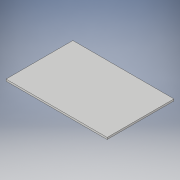
# Autodesk Inventor part: basic side
Saved by Autodesk Inventor 2018 (Build 220112000, 112)
## iProperties
Created: 2018-05-14
Part Number: basic side
Material: Generic
Document SubType Name: Modeling
Designer: Administrator
Density: 1 g/cm^3
Appearance: Default
Author: Administrator
Autodesk Inventor part; units mm, degrees
ref_plane "YZ Plane" through (0, 0, 0) normal (1, 0, 0) x (0, 1, 0)
ref_plane "XZ Plane" through (0, 0, 0) normal (0, 1, 0) x (-1, 0, 0)
ref_plane "XY Plane" through (0, 0, 0) normal (0, 0, 1) x (1, 0, 0)
sketch "Sketch1" plane through (0, 0, 0) normal (0, 0, 1) x (1, 0, 0)
  line L0 (0, 0) -> (355.6, 0)
  line L1 (355.6, 0) -> (355.6, 152.4)
  line L2 (355.6, 152.4) -> (0, 152.4)
  line L3 (0, 152.4) -> (0, 0)
  circle A0 centre (177.8, 76.2) radius 12.7
  circle A1 centre (279.4, 76.2) radius 12.7
  circle A2 centre (76.2, 76.2) radius 12.7
  dimension "d2" = 25.4
  dimension "d3" = 25.4
  dimension "d5" = 25.4
  dimension "d8" = 355.6
  dimension "d9" = 152.4
  dimension "d10" = 101.6
  dimension "d11" = 101.6
  constraints: 8 end point, 3 centre point, 2 parallel, 1 horizontal, 1 perpendicular
  measures "d2" diameter of A0
  measures "d3" diameter of A1
  measures "d5" diameter of A2
  measures "d8" distance of L1.end L2.end
  measures "d9" distance of L0.end L1.end
  measures "d10" distance of A0.centre A2.centre
  measures "d11" distance of A0.centre A1.centre
extrude "Extrusion1" add sketch "Sketch1" along normal blind 12.7
sketch "Sketch2" plane through (0, 0, 12.7) normal (0, 0, 1) x (1, 0, 0)
  line L0 (0, 152.4) -> (0, 0) projected
  line L1 (0, 152.4) -> (0, 165.1)
  line L2 (0, 165.1) -> (-12.7, 165.1)
  line L3 (-12.7, 165.1) -> (-12.7, -12.7)
  line L4 (-12.7, -12.7) -> (0, -12.7)
  line L5 (0, -12.7) -> (0, 0)
  line L6 (355.6, 152.4) -> (0, 152.4) projected
  line L7 (0, 0) -> (0, 152.4)
  line L8 (0, 165.1) -> (355.6, 165.1)
  line L9 (355.6, 0) -> (355.6, 152.4) projected
  line L10 (355.6, 165.1) -> (355.6, 152.4)
  line L11 (355.6, 152.4) -> (0, 152.4)
  line L12 (355.6, 165.1) -> (368.3, 165.1)
  line L13 (368.3, 165.1) -> (368.3, -12.7)
  line L14 (368.3, -12.7) -> (355.6, -12.7)
  line L15 (355.6, -12.7) -> (355.6, 0)
  line L16 (0, -12.7) -> (355.6, -12.7)
  line L17 (0, 0) -> (355.6, 0) projected
  line L18 (0, 0) -> (355.6, 0)
  dimension "d14" = 12.7
  dimension "d15" = 12.7
  dimension "d16" = 177.8
  dimension "d17" = 12.7
  dimension "d18" = 177.8
  constraints: 30 end point, 9 perpendicular, 2 collinear, 2 point on line, 1 horizontal, 1 vertical
  measures "d14" distance of L0.start L1.end
  measures "d15" distance of L1.end L2.end
  measures "d16" distance of L2.end L3.end
  measures "d17" distance of L8.end L12.end
  measures "d18" distance of L12.end L13.end
extrude "Extrusion2" add sketch "Sketch2" against normal blind 241.3 contours L1 L8 L10 L6
extrude "Extrusion3" add sketch "Sketch2" against normal blind 241.3 contours L0 L5 L4 L3 L2 L1
extrude "Extrusion4" add sketch "Sketch2" against normal blind 241.3 contours L17 L15 L16 L5
extrude "Extrusion5" add sketch "Sketch2" against normal blind 241.3 contours L10 L12 L13 L14 L15 L9
sketch "Sketch3" plane through (368.3, -12.7, 12.7) normal (1, 0, 0) x (0, 0, -1)
  line L0 (241.3, 165.1) -> (241.3, 12.7) projected
  line L1 (241.3, 12.7) -> (241.3, 38.1)
  line L2 (241.3, 38.1) -> (215.9, 38.1)
  line L3 (215.9, 38.1) -> (215.9, 107.95)
  line L4 (215.9, 107.95) -> (241.3, 107.95)
  point P0 (12.7, 12.7)
  dimension "d27" = 25.4
  dimension "d28" = 25.4
  dimension "d29" = 69.85
  constraints: 8 end point, 2 perpendicular, 2 point on line, 1 horizontal
  measures "d27" distance of L0.end L1.end
  measures "d28" distance of L1.end L2.end
  measures "d29" distance of L2.end L3.end
extrude "Extrusion6" cut sketch "Sketch3" against normal blind 212.725
move faces "Move1" translate (-6.35, 0, 0) faces at (368.3, 82.55, -59.2667)
move faces "Move2" translate (0, -6.35, 0) faces at (237.0667, 165.1, -67.7333)
move faces "Move3" translate (0, 6.35, 0) faces at (112.1833, -12.7, -67.7333)
move faces "Move4" translate (6.35, 0, 0) faces at (-12.7, 103.7167, -67.7333)
move faces "Move5" translate (0, 0, -6.35) faces at (178.3103, 135.4358, 12.7)
sketch "Sketch4" plane through (-6.35, -6.35, 6.35) normal (0, 0, 1) x (1, 0, 0)
  circle A0 centre (184.15, 82.55) radius 12.7 projected
  line L0 (184.15, 82.55) -> (151.13, 82.55)
  line L1 (151.13, 82.55) -> (151.13, 120.65)
  line L2 (151.13, 82.55) -> (151.13, 44.45)
  line L3 (184.15, 82.55) -> (217.17, 82.55)
  line L4 (217.17, 82.55) -> (217.17, 120.65)
  line L5 (217.17, 82.55) -> (217.17, 44.45)
  circle A1 centre (285.75, 82.55) radius 12.7 projected
  line L6 (285.75, 82.55) -> (252.73, 82.55)
  line L7 (252.73, 82.55) -> (252.73, 120.65)
  line L8 (252.73, 82.55) -> (252.73, 44.45)
  line L9 (285.75, 82.55) -> (318.77, 82.55)
  line L10 (318.77, 82.55) -> (318.77, 120.65)
  line L11 (318.77, 82.55) -> (318.77, 44.45)
  circle A2 centre (82.55, 82.55) radius 12.7 projected
  line L12 (82.55, 82.55) -> (115.57, 82.55)
  line L13 (115.57, 82.55) -> (115.57, 120.65)
  line L14 (115.57, 82.55) -> (115.57, 44.45)
  line L15 (82.55, 82.55) -> (49.53, 82.55)
  line L16 (49.53, 82.55) -> (49.53, 120.65)
  line L17 (49.53, 82.55) -> (49.53, 44.45)
  circle A3 centre (151.13, 120.65) radius 3.175
  circle A4 centre (217.17, 120.65) radius 3.175
  circle A5 centre (151.13, 44.45) radius 3.175
  circle A6 centre (217.17, 44.45) radius 3.175
  circle A7 centre (49.53, 120.65) radius 3.175
  circle A8 centre (49.53, 44.45) radius 3.175
  circle A9 centre (115.57, 120.65) radius 3.175
  circle A10 centre (115.57, 44.45) radius 3.175
  circle A11 centre (252.73, 120.65) radius 3.175
  circle A12 centre (318.77, 120.65) radius 3.175
  circle A13 centre (252.73, 44.45) radius 3.175
  circle A14 centre (318.77, 44.45) radius 3.175
  point P0 (6.35, 6.35)
  dimension "d47" = 33.02
  dimension "d48" = 38.1
  dimension "d49" = 38.1
  dimension "d50" = 33.02
  dimension "d51" = 38.1
  dimension "d52" = 38.1
  dimension "d53" = 33.02
  dimension "d54" = 33.02
  dimension "d55" = 33.02
  dimension "d56" = 33.02
  dimension "d57" = 38.1
  dimension "d58" = 38.1
  dimension "d59" = 38.1
  dimension "d60" = 38.1
  dimension "d61" = 38.1
  dimension "d62" = 38.1
  dimension "d63" = 38.1
  dimension "d64" = 38.1
  dimension "d65" = 6.35
  dimension "d66" = 6.35
  dimension "d67" = 6.35
  dimension "d68" = 6.35
  dimension "d69" = 6.35
  dimension "d70" = 6.35
  dimension "d71" = 6.35
  dimension "d72" = 6.35
  dimension "d73" = 6.35
  dimension "d74" = 6.35
  dimension "d75" = 6.35
  dimension "d76" = 6.35
  constraints: 36 end point, 12 centre point, 12 coincident, 7 perpendicular, 6 horizontal, 5 vertical
  measures "d47" distance of L0.start L0.end
  measures "d48" distance of L0.end L1.end
  measures "d49" distance of L0.end L2.end
  measures "d50" distance of L0.start L3.end
  measures "d51" distance of L3.end L4.end
  measures "d52" distance of L3.end L5.end
  measures "d53" distance of L6.start L6.end
  measures "d54" distance of L6.start L9.end
  measures "d55" distance of L12.start L12.end
  measures "d56" distance of L12.start L15.end
  measures "d57" distance of L12.end L13.end
  measures "d58" distance of L12.end L14.end
  measures "d59" distance of L15.end L17.end
  measures "d60" distance of L15.end L16.end
  measures "d61" distance of L6.end L7.end
  measures "d62" distance of L9.end L10.end
  measures "d63" distance of L9.end L11.end
  measures "d64" distance of L6.end L8.end
  measures "d65" diameter of A3
  measures "d66" diameter of A4
  measures "d67" diameter of A5
  measures "d68" diameter of A6
  measures "d69" diameter of A7
  measures "d70" diameter of A8
  measures "d71" diameter of A9
  measures "d72" diameter of A10
  measures "d73" diameter of A11
  measures "d74" diameter of A12
  measures "d75" diameter of A13
  measures "d76" diameter of A14
extrude "Extrusion7" cut sketch "Sketch4" against normal blind 88.9 contours A3 | A4 | A5 | A6 | A7 | A8 | A9 | A10 | A11 | A12 | A13 | A14
sketch "Sketch5" plane through (361.95, 25.4, -203.2) normal (1, 0, 0) x (0, 0, -1)
  line L0 (0, 0) -> (0, 69.85) projected
  line L1 (0, 0) -> (0, 63.5)
  line L2 (0, 69.85) -> (0, 0) projected
  line L3 (0, 63.5) -> (-38.1, 63.5)
  circle A0 centre (-38.1, 63.5) radius 3.175
  circle A1 centre (-46.99, 63.5) radius 3.175
  circle A2 centre (-55.88, 63.5) radius 3.175
  circle A3 centre (-64.77, 63.5) radius 3.175
  circle A4 centre (-73.66, 63.5) radius 3.175
  circle A5 centre (-38.1, 72.39) radius 3.175
  circle A6 centre (-46.99, 72.39) radius 3.175
  circle A7 centre (-55.88, 72.39) radius 3.175
  circle A8 centre (-64.77, 72.39) radius 3.175
  circle A9 centre (-73.66, 72.39) radius 3.175
  circle A10 centre (-38.1, 81.28) radius 3.175
  circle A11 centre (-46.99, 81.28) radius 3.175
  circle A12 centre (-55.88, 81.28) radius 3.175
  circle A13 centre (-64.77, 81.28) radius 3.175
  circle A14 centre (-73.66, 81.28) radius 3.175
  point P0 (-203.2, -25.4)
  dimension "d79" = 63.5
  dimension "d80" = 38.1
  dimension "d81" = 6.35
  dimension "d84" = 8.89
  dimension "d87" = 8.89
  constraints: 15 centre point, 4 end point, 2 horizontal, 1 coincident, 1 point on line, 1 vertical, 28 other
  measures "d79" distance of L0.start L1.end
  measures "d80" distance of L1.end L3.end
  measures "d81" diameter of A0
  measures "d84" distance of A0.centre A1.centre
  measures "d87" distance of A0.centre A5.centre
extrude "Extrusion8" cut sketch "Sketch5" against normal blind 39.6875
extrude "Extrusion9" cut sketch "Sketch5" against normal blind 530.225
move faces "Move6" translate (0, 0, 133.35) faces at (155.0676, 140.7506, 0)
move faces "Move7" translate (0, -47.625, 0) faces at (237.0667, 0, -71.9667)
move faces "Move8" translate (-6.35, 0, 0) faces at (361.95, 80.1801, -37.9191)
move faces "Move9" translate (6.35, 0, 0) faces at (-6.35, 80.1801, -37.9191)
body "Solid1"
